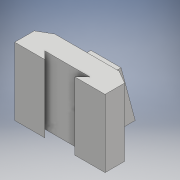
# Autodesk Inventor part: P3-15
Saved by Autodesk Inventor 2017 (Build 210142000, 142)
## iProperties
Created: 2017-02-13
Part Number: P3-15
Material: Generic
Document SubType Name: Modeling
Designer: Schaffel
Density: 1 g/cm^3
Appearance: Default
Author: Schaffel
Autodesk Inventor part; units mm, degrees
ref_plane "YZ Plane" through (0, 0, 0) normal (1, 0, 0) x (0, 1, 0)
ref_plane "XZ Plane" through (0, 0, 0) normal (0, 1, 0) x (-1, 0, 0)
ref_plane "XY Plane" through (0, 0, 0) normal (0, 0, 1) x (1, 0, 0)
sketch "Sketch1" plane through (0, 0, 0) normal (0, 0, 1) x (1, 0, 0)
  line L0 (0, 0) -> (20, 0)
  line L1 (20, 0) -> (15, 5)
  line L2 (15, 5) -> (45, 5)
  line L3 (45, 5) -> (40, 0)
  line L4 (40, 0) -> (60, 0)
  line L5 (60, 0) -> (60, 13)
  line L6 (0, 0) -> (0, 13)
  line L7 (20, 24.547) -> (20, 40)
  line L8 (20, 40) -> (40, 40)
  line L9 (40, 40) -> (40, 24.547)
  line L10 (60, 13) -> (40, 24.547)
  line L11 (20, 24.547) -> (0, 13)
  constraints: 24 end point, 4 perpendicular, 2 horizontal, 1 parallel, 1 vertical
extrude "Extrusion1" add sketch "Sketch1" along normal blind 45
sketch "Sketch2" plane through (0, 0, 45) normal (0, 0, 1) x (1, 0, 0)
  line L0 (20, 24.547) -> (0, 13) projected
  line L1 (8.6603, 18) -> (51.3397, 18)
  line L2 (60, 13) -> (40, 24.547) projected
  line L3 (8.6603, 18) -> (20, 24.547)
  line L4 (20, 40) -> (20, 24.547) projected
  line L5 (20, 24.547) -> (20, 40)
  line L6 (20, 40) -> (40, 40)
  line L7 (40, 40) -> (40, 24.547)
  line L8 (40, 24.547) -> (40, 40) projected
  line L9 (40, 24.547) -> (51.3397, 18)
  point P0 (0, 0)
  constraints: 12 end point, 3 point on line, 2 perpendicular, 1 collinear, 1 horizontal
extrude "Extrusion2" cut sketch "Sketch2" against normal blind 10
sketch "Sketch3" plane through (40, 24.547, 0) normal (1, 0, 0) x (0, 0, -1)
  line L0 (0, 0) -> (0, 15.453) projected
  line L1 (0, 15.453) -> (37.2699, 15.453) construction
  line L2 (-35, 0) -> (-35, 15.453) projected
  line L3 (-35, 15.453) -> (0, 15.453)
  line L4 (0, 15.453) -> (-35, 6.0748)
  line L5 (-35, 6.0748) -> (-35, 15.453)
  point P0 (0, -24.547)
  constraints: 8 end point, 2 perpendicular, 1 horizontal
extrude "Extrusion3" cut sketch "Sketch3" against normal blind 20
sketch "Sketch4" plane through (60, 0, 0) normal (1, 0, 0) x (0, 0, -1)
  line L0 (0, 18) -> (-10, 18)
  line L1 (-10, 18) -> (-10, 24.547)
  line L2 (0, 24.547) -> (-35, 24.547) projected
  line L3 (0, 24.547) -> (0, 40) projected
  line L4 (-10, 24.547) -> (0, 24.547)
  line L5 (0, 24.547) -> (0, 18)
  point P0 (0, 0)
  constraints: 8 end point, 2 horizontal, 2 perpendicular, 1 point on line
extrude "Extrusion4" cut sketch "Sketch4" against normal blind 20
sketch "Sketch5" plane through (0, 0, 0) normal (-1, 0, 0) x (0, 0, 1)
  line L0 (10, 18) -> (10, 24.547) projected
  line L1 (10, 18) -> (10, 24.547)
  line L2 (0, 24.547) -> (35, 24.547) projected
  line L3 (10, 24.547) -> (0, 24.547)
  line L4 (0, 24.547) -> (0, 18)
  line L5 (0, 24.547) -> (0, 13) projected
  line L6 (0, 18) -> (10, 18) projected
  line L7 (10, 18) -> (0, 18)
  point P0 (0, 0)
  constraints: 8 end point, 3 collinear, 1 point on line
extrude "Extrusion5" cut sketch "Sketch5" against normal blind 20
body "Solid1"
